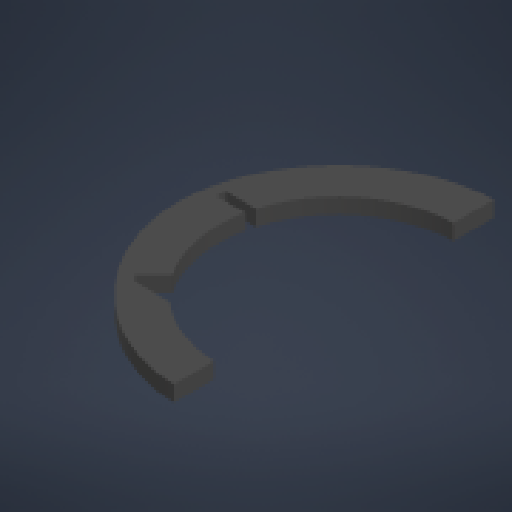
# Autodesk Inventor part: Back_back_aligner
Saved by Autodesk Inventor 2023 (Build 270158000, 158)
## iProperties
Created: 2023-05-09
Part Number: Back_back_aligner
Material: Generic
Document SubType Name: Modeling
Designer: szykr
Density: 1 g/cm^3
Appearance: Rubber - Black
Author: szykr
Autodesk Inventor part; units mm, degrees
ref_plane "YZ Plane" through (0, 0, 0) normal (1, 0, 0) x (0, 1, 0)
ref_plane "XZ Plane" through (0, 0, 0) normal (0, 1, 0) x (-1, 0, 0)
ref_plane "XY Plane" through (0, 0, 0) normal (0, 0, 1) x (1, 0, 0)
sketch "Sketch1" plane through (0, 0, 0) normal (0, 1, 0) x (-1, 0, 0)
  line L0 (-40, -22.2559) -> (-17.5965, -22.2559) projected
  spline S0 degree 3 poles (-17.5965, -22.2559) (-16.6656, -23.0054) (-15.6914, -23.7008) (-11.4898, -26.3394) (-7.9349, -27.7425) (-1.802, -28.767) (1.7129, -29.0153) (9.4587, -27.1875) (12.7711, -25.6792) (16.3694, -23.2064) (16.9921, -22.7425) (17.5965, -22.2559) knots 1.921938 1.921938 1.921938 1.921938 2.28002 2.28002 3.408568 3.408568 4.146561 4.146561 4.751486 4.751486 4.882227 4.882227 4.882227 4.882227 projected
  line L1 (17.5965, -22.2559) -> (40, -22.2559) projected
  line L2 (40, -22.2559) -> (40, -16.3077) projected
  line L3 (40, -16.3077) -> (23.2525, -16.3077) projected
  spline S1 degree 3 poles (23.2525, -16.3077) (24.6957, -14.3166) (25.8988, -12.1536) (28.0747, -6.71) (28.7719, -3.3404) (28.7749, 0.0586) knots 0.307224 0.307224 0.307224 0.307224 1.04533 1.04533 2.067491 2.067491 2.067491 2.067491 projected
  spline S2 degree 3 poles (28.7749, 0.0586) (28.7778, 3.3432) (28.1322, 6.6023) (25.6023, 13.1892) (23.5632, 16.432) (18.302, 22.1753) (15.0141, 24.6102) (8.1089, 27.8149) (4.5799, 28.7211) (-2.7873, 29.0129) (-6.0815, 28.2969) (-12.2596, 26.1389) (-15.5213, 24.2237) (-21.3931, 19.1817) (-23.9297, 15.9754) (-27.394, 9.1373) (-28.4362, 5.5845) (-28.8291, 0.2785) (-28.786, -1.3758) (-28.2317, -5.891) (-27.4068, -8.6862) (-25.3769, -13.0646) (-24.3891, -14.7396) (-23.2525, -16.3077) knots 0 0 0 0 0.985401 0.985401 2.113862 2.113862 3.316195 3.316195 4.394104 4.394104 5.528611 5.528611 7.023718 7.023718 8.634698 8.634698 10.102311 10.102311 10.775364 10.775364 11.944404 11.944404 12.727759 12.727759 12.727759 12.727759 projected
  line L4 (-23.2525, -16.3077) -> (-40, -16.3077) projected
  line L5 (-40, -16.3077) -> (-40, -22.2559) projected
  circle A0 centre (0, 0.0832) radius 23 projected
  line L6 (0.75, 28.2736) -> (0.75, 23.0832) projected
  line L7 (19.2521, 12.9144) -> (23.1341, 16.806) projected
  line L8 (22.3297, -4.6807) -> (27.9307, -4.6807) projected
  line L9 (27.9307, -6.177) -> (22.3297, -6.177) projected
  line L10 (0.75, -22.9168) -> (0.75, -28.7163) projected
  line L11 (19.2521, 12.9144) -> (19.1539, 12.8161)
  line L12 (26.9025, -14.3077) -> (42, -14.3077)
  line L13 (42, -14.3077) -> (42, -24.2559)
  line L14 (42, -24.2559) -> (18.2892, -24.2559)
  line L15 (-18.2892, -24.2559) -> (-42, -24.2559)
  line L16 (-42, -24.2559) -> (-42, -14.3077)
  line L17 (-42, -14.3077) -> (-26.9025, -14.3077)
  line L18 (22.3035, 16.9291) -> (22.8338, 16.4001) projected
  line L19 (22.3035, 16.9291) -> (21.7732, 17.4581) projected
  line L20 (21.7732, 17.4581) -> (15.0702, 17.4581)
  line L21 (0.75, 28.2736) -> (0.75, 30.8725)
  line L22 (22.3297, -6.177) -> (22.1316, -6.177)
  line L23 (27.9307, -5.4288) -> (27.9307, -4.6807) projected
  line L24 (27.9307, -5.4288) -> (27.9307, -6.177) projected
  line L25 (22.1031, -6.277) -> (27.9768, -6.277)
  line L26 (28.0307, -4.5807) -> (28.0307, -6.277)
  line L27 (28.0307, -6.277) -> (27.9768, -6.277)
  line L28 (28.0307, -4.5807) -> (22.5222, -4.5807)
  arc A1 (18.2892, -24.2559) -> (26.9025, -14.3077) centre (-2.2893, 2.264) ccw
  line L29 (0.75, -28.7163) -> (0.75, -30.7052)
  line L30 (0.75, 23.0832) -> (0.75, 23.071)
  line L31 (0.75, -22.9168) -> (0.75, -22.9046)
  spline S3 degree 5 poles (-26.9025, -14.3077) (-27.429, -13.3679) (-27.9159, -12.406) (-28.3615, -11.4239) (-29.4514, -8.7146) (-30.2109, -5.8891) (-30.5495, -4.0723) (-30.9282, -0.387) (-30.677, 3.3095) (-30.3948, 5.1476) (-29.5444, 8.755) (-28.1523, 12.1901) (-27.3327, 13.8493) (-25.462, 17.0353) (-23.1617, 19.9263) (-21.9138, 21.288) (-19.2364, 23.8311) (-16.2309, 25.977) (-14.6542, 26.9424) (-11.1856, 28.736) (-7.4774, 29.9652) (-5.4735, 30.4505) (-0.9788, 31.1008) (3.5628, 30.8183) (6.0146, 30.3783) (10.7855, 29.0025) (15.1886, 26.7031) (17.271, 25.3465) (21.1567, 22.2584) (24.4033, 18.5051) (25.8467, 16.4825) (28.3392, 12.1746) (29.9378, 7.461) (30.4933, 5.0225) (30.7772, 2.5393) (30.7749, 0.0568) knots 0 0 0 0 0 0 0.04843 0.04843 0.04843 0.131166 0.131166 0.131166 0.214396 0.214396 0.214396 0.297313 0.297313 0.297313 0.380087 0.380087 0.380087 0.462936 0.462936 0.462936 0.55515 0.55515 0.55515 0.666218 0.666218 0.666218 0.77732 0.77732 0.77732 0.888384 0.888384 0.888384 1 1 1 1 1 1
  spline S4 degree 5 poles (30.7749, 0.0568) (30.7726, -2.951) (30.349, -5.9587) (29.5343, -8.8867) (28.3726, -11.6837) (26.9025, -14.3077) knots 0 0 0 0 0 0 1 1 1 1 1 1
  spline S5 degree 5 poles (18.2892, -24.2559) (16.1748, -25.8838) (13.8947, -27.2963) (11.4761, -28.469) (6.8505, -30.1183) (1.9949, -30.776) (-0.231, -30.8531) (-4.0328, -30.578) (-7.7292, -29.6857) (-9.2444, -29.2094) (-12.0661, -28.1171) (-14.7351, -26.6935) (-15.965, -25.9461) (-17.1511, -25.1321) (-18.2892, -24.2559) knots 0 0 0 0 0 0 0.337839 0.337839 0.337839 0.617671 0.617671 0.617671 0.818155 0.818155 0.818155 1 1 1 1 1 1
  point P0 (0, 0)
  point P1 (22.7814, 16.4524)
  dimension "d0" = 2
  dimension "d1" = 0.1
  dimension "d2" = 0.1
  dimension "d3" = 0.1
  constraints: 34 end point, 6 parallel, 4 collinear, 3 vertical, 2 point on circle, 1 centre point, 1 horizontal, 24 other
  measures "d1" distance between parallel lines of L9 L25
  measures "d2" distance between parallel lines of L23 L26
  measures "d3" distance between parallel lines of L8 L28
extrude "Extrusion1" add sketch "Sketch1" along normal blind 3 contours L10 L31 A0 L25 S1 L3 A1 L1 S0 | S0 L1 A1 S5 L29 L10 | L21 S3 S4 A1 L3 S1 L27 L26 S2 | S2 L7 L18 L19 L20 A0 L30 L6 L21 | S2 S1 L26 L28 A0 L11 L7
equation "\"d2\" = slack"
equation "\"d3\" = slack"
equation "\"slack\" = 0.1"
body "Solid1"
